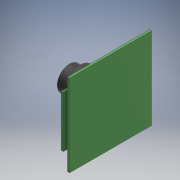
# Autodesk Inventor part: learnbotCamara
Saved by Autodesk Inventor 2017 (Build 210142000, 142)
## iProperties
Part Number: learnbotCamara
Material: Genérico
Document SubType Name: Modeling
Designer: rober
Density: 1 g/cm^3
Appearance: Valor por defecto
Author: rober
Autodesk Inventor part; units mm, degrees
ref_plane "YZ Plane" through (0, 0, 0) normal (1, 0, 0) x (0, 1, 0)
ref_plane "XZ Plane" through (0, 0, 0) normal (0, 1, 0) x (-1, 0, 0)
ref_plane "XY Plane" through (0, 0, 0) normal (0, 0, 1) x (1, 0, 0)
sketch "Boceto1" plane through (0, 0, 0) normal (0, 0, 1) x (1, 0, 0)
  line L0 (-1.6, 1.6) -> (-1.6, 1.2)
  line L1 (-1.1, 1.2) -> (-1.1, 2.8)
  line L2 (-1.1, 2.8) -> (-0.9, 2.8)
  line L3 (-0.9, 2.8) -> (-0.9, 1.2)
  line L4 (-0.2, 0.75) -> (-0.2, 3.25)
  line L5 (-0.9, 2.6) -> (-0.2, 2.6)
  line L6 (-0.2, 3.25) -> (0, 3.25)
  line L7 (0, 0) -> (0, 4)
  line L8 (-0.2, 0.75) -> (0, 0.75)
  line L9 (-1.1, 1) -> (-1.1, 1.2)
  line L10 (-0.9, 1.2) -> (-0.9, 1)
  line L11 (-1.1, 1) -> (-0.9, 1)
  line L12 (-1.6, 1.2) -> (-1.1, 1.2)
  line L13 (-0.9, 1.2) -> (-0.2, 1.2)
  line L14 (-1.1, 2.6) -> (-1.6, 2.6)
  line L15 (0.3, 0) -> (0.3, 4)
  line L16 (0, 0) -> (0.1, 0)
  line L17 (0.1, 0) -> (0.1, 4)
  line L18 (0.1, 4) -> (0, 4)
  line L19 (0.3, 0) -> (0.4, 0)
  line L20 (0.4, 0) -> (0.4, 4)
  line L21 (0.4, 4) -> (0.3, 4)
  line L22 (-1.6, 1.6) -> (-1.5, 1.6)
  line L23 (-1.5, 1.6) -> (-1.5, 2.2)
  line L24 (-1.5, 2.2) -> (-1.6, 2.2)
  line L25 (-1.6, 2.2) -> (-1.6, 2.6)
  constraints: 52 end point, 6 point on line
extrude "Extrusión1" add sketch "Boceto1" along normal blind 4 contours L7 L18 L17 L16 | L15 L21 L20 L19
sketch "Boceto2" plane through (0, 0, 0) normal (-1, 0, 0) x (0, 0, 1)
  line L0 (0, 4) -> (0, 0) projected
  line L1 (0, 0) -> (4, 0) projected
  line L2 (4, 4) -> (4, 0) projected
  line L3 (0, 4) -> (4, 4) projected
  line L4 (0, 4) -> (4, 4)
  line L5 (4, 0) -> (0, 0)
  line L6 (0, 0) -> (0, 4)
  circle A0 centre (2, 2) radius 0.8
  circle A1 centre (2, 2) radius 0.35
  circle A2 centre (2, 2) radius 0.6
  line L7 (1.4, 1.2) -> (1.4, 1.4708)
  line L8 (1.4, 2.5292) -> (1.4, 2.8)
  line L9 (2.6, 2.8) -> (2.6, 2.5292)
  line L10 (2.6, 1.4708) -> (2.6, 1.2)
  line L11 (2.4395, 1.2) -> (1.5605, 1.2)
  line L12 (1.4, 1.2) -> (1.9377, 0.7718)
  line L13 (2.0623, 0.7718) -> (2.6, 1.2)
  circle A3 centre (2, 3.15) radius 0.1
  circle A4 centre (2, 0.85) radius 0.1
  line L14 (1.5605, 1.2) -> (1.9218, 0.9123)
  line L15 (2.4395, 1.2) -> (2.0782, 0.9123)
  line L16 (2.4395, 2.8) -> (1.5605, 2.8)
  line L17 (1.5605, 2.8) -> (1.9218, 3.0877)
  line L18 (2.4395, 2.8) -> (2.0782, 3.0877)
  line L19 (1.4, 2.8) -> (1.9377, 3.2282)
  line L20 (2.0623, 3.2282) -> (2.6, 2.8)
  line L21 (0.75, 0) -> (0.75, 4)
  line L22 (0.75, 4) -> (3.25, 4)
  line L23 (3.25, 4) -> (3.25, 0)
  line L24 (4, 0) -> (4, 4)
  constraints: 42 end point, 12 point on circle, 5 centre point, 4 point on line
extrude "Extrusión2" cut sketch "Boceto2" against normal blind 0.2 contours L3 L21 L1 L0 | L3 L2 L1 L23
sketch "Boceto3" plane through (0, 0, 0.75) normal (-1, 0, 0) x (0, 0, 1)
  line L0 (-0.75, 4) -> (3.25, 4)
  line L1 (3.25, 0) -> (-0.75, 0)
  line L2 (-0.75, 0) -> (-0.75, 4)
  circle A0 centre (1.25, 2) radius 0.8
  circle A1 centre (1.25, 2) radius 0.35
  circle A2 centre (1.25, 2) radius 0.6
  line L3 (0.65, 1.2) -> (0.65, 1.4708)
  line L4 (0.65, 2.5292) -> (0.65, 2.8)
  line L5 (1.85, 2.8) -> (1.85, 2.5292)
  line L6 (1.85, 1.4708) -> (1.85, 1.2)
  line L7 (1.6895, 1.2) -> (0.8105, 1.2)
  line L8 (0.65, 1.2) -> (1.1877, 0.7718)
  line L9 (1.3123, 0.7718) -> (1.85, 1.2)
  circle A3 centre (1.25, 3.15) radius 0.1
  circle A4 centre (1.25, 0.85) radius 0.1
  line L10 (0.8105, 1.2) -> (1.1718, 0.9123)
  line L11 (1.6895, 1.2) -> (1.3282, 0.9123)
  line L12 (1.6895, 2.8) -> (0.8105, 2.8)
  line L13 (0.8105, 2.8) -> (1.1718, 3.0877)
  line L14 (1.6895, 2.8) -> (1.3282, 3.0877)
  line L15 (0.65, 2.8) -> (1.1877, 3.2282)
  line L16 (1.3123, 3.2282) -> (1.85, 2.8)
  line L17 (0, 0) -> (0, 4)
  line L18 (0, 4) -> (2.5, 4)
  line L19 (2.5, 4) -> (2.5, 0)
  line L20 (3.25, 0) -> (3.25, 4)
  line L21 (0, 4) -> (0, 0) projected
  line L22 (0, 0) -> (2.5, 0) projected
  line L23 (2.5, 0) -> (2.5, 4) projected
  line L24 (0, 4) -> (2.5, 4) projected
  constraints: 42 end point, 12 point on circle, 5 centre point, 4 point on line
extrude "Extrusión3" add sketch "Boceto3" along normal blind 0.2 contours A0 | A0 L12 L14 A3 L16 L5 | L6 L9 A4 L11 L7 A0 | A0 L4 L15 A3 L13 L12 | L7 L10 A4 L8 L3 A0 | A3 | A4 | A1 | A2
sketch "Boceto4" plane through (-0.2, 0, 0.75) normal (-1, 0, 0) x (0, 0, 1)
  line L0 (-0.75, 4) -> (3.25, 4)
  line L1 (3.25, 0) -> (-0.75, 0)
  line L2 (-0.75, 0) -> (-0.75, 4)
  circle A0 centre (1.25, 2) radius 0.8
  circle A1 centre (1.25, 2) radius 0.35
  circle A2 centre (1.25, 2) radius 0.6
  line L3 (0.65, 1.2) -> (0.65, 1.4708)
  line L4 (0.65, 2.5292) -> (0.65, 2.8)
  line L5 (1.85, 2.8) -> (1.85, 2.5292)
  line L6 (1.85, 1.4708) -> (1.85, 1.2)
  line L7 (1.6895, 1.2) -> (0.8105, 1.2)
  line L8 (0.65, 1.2) -> (1.1877, 0.7718)
  line L9 (1.3123, 0.7718) -> (1.85, 1.2)
  circle A3 centre (1.25, 3.15) radius 0.1
  circle A4 centre (1.25, 0.85) radius 0.1
  line L10 (0.8105, 1.2) -> (1.1718, 0.9123)
  line L11 (1.6895, 1.2) -> (1.3282, 0.9123)
  line L12 (1.6895, 2.8) -> (0.8105, 2.8)
  line L13 (0.8105, 2.8) -> (1.1718, 3.0877)
  line L14 (1.6895, 2.8) -> (1.3282, 3.0877)
  line L15 (0.65, 2.8) -> (1.1877, 3.2282)
  line L16 (1.3123, 3.2282) -> (1.85, 2.8)
  line L17 (0, 0) -> (0, 4)
  line L18 (0, 4) -> (2.5, 4)
  line L19 (2.5, 4) -> (2.5, 0)
  line L20 (3.25, 0) -> (3.25, 4)
  line L21 (1.6895, 2.8) -> (0.8105, 2.8) projected
  line L22 (0.8105, 2.8) -> (1.1718, 3.0877) projected
  arc A5 (1.1718, 3.0877) -> (1.3282, 3.0877) centre (1.25, 3.15) ccw projected
  line L23 (1.3282, 3.0877) -> (1.6895, 2.8) projected
  line L24 (1.6895, 1.2) -> (1.3282, 0.9123) projected
  arc A6 (1.3282, 0.9123) -> (1.1718, 0.9123) centre (1.25, 0.85) ccw projected
  line L25 (1.1718, 0.9123) -> (0.8105, 1.2) projected
  line L26 (0.8105, 1.2) -> (1.6895, 1.2) projected
  line L27 (0.65, 1.2) -> (1.1877, 0.7718) projected
  arc A7 (1.1877, 0.7718) -> (1.3123, 0.7718) centre (1.25, 0.85) ccw projected
  line L28 (1.3123, 0.7718) -> (1.85, 1.2) projected
  line L29 (1.85, 1.2) -> (1.85, 1.4708) projected
  arc A8 (1.85, 1.4708) -> (1.85, 2.5292) centre (1.25, 2) ccw projected
  line L30 (1.85, 2.5292) -> (1.85, 2.8) projected
  line L31 (1.85, 2.8) -> (1.3123, 3.2282) projected
  arc A9 (1.3123, 3.2282) -> (1.1877, 3.2282) centre (1.25, 3.15) ccw projected
  line L32 (1.1877, 3.2282) -> (0.65, 2.8) projected
  line L33 (0.65, 2.8) -> (0.65, 2.5292) projected
  arc A10 (0.65, 2.5292) -> (0.65, 1.4708) centre (1.25, 2) ccw projected
  line L34 (0.65, 1.4708) -> (0.65, 1.2) projected
  point P0 (-0.75, 0)
  constraints: 42 end point, 12 point on circle, 5 centre point, 4 point on line
extrude "Extrusión4" add sketch "Boceto4" along normal blind 0.7 contours A1 | A2
sketch "Boceto5" plane through (-0.9, 2, 2) normal (-1, 0, 0) x (0, 0, 1)
  line L0 (-2, 2) -> (2, 2)
  line L1 (2, -2) -> (-2, -2)
  line L2 (-2, -2) -> (-2, 2)
  circle A0 centre (0, 0) radius 0.8
  circle A1 centre (0, 0) radius 0.35
  circle A2 centre (0, 0) radius 0.6
  line L3 (-0.6, -0.8) -> (-0.6, -0.5292)
  line L4 (-0.6, 0.5292) -> (-0.6, 0.8)
  line L5 (0.6, 0.8) -> (0.6, 0.5292)
  line L6 (0.6, -0.5292) -> (0.6, -0.8)
  line L7 (0.4395, -0.8) -> (-0.4395, -0.8)
  line L8 (-0.6, -0.8) -> (-0.0623, -1.2282)
  line L9 (0.0623, -1.2282) -> (0.6, -0.8)
  circle A3 centre (0, 1.15) radius 0.1
  circle A4 centre (0, -1.15) radius 0.1
  line L10 (-0.4395, -0.8) -> (-0.0782, -1.0877)
  line L11 (0.4395, -0.8) -> (0.0782, -1.0877)
  line L12 (0.4395, 0.8) -> (-0.4395, 0.8)
  line L13 (-0.4395, 0.8) -> (-0.0782, 1.0877)
  line L14 (0.4395, 0.8) -> (0.0782, 1.0877)
  line L15 (-0.6, 0.8) -> (-0.0623, 1.2282)
  line L16 (0.0623, 1.2282) -> (0.6, 0.8)
  line L17 (-1.25, -2) -> (-1.25, 2)
  line L18 (-1.25, 2) -> (1.25, 2)
  line L19 (1.25, 2) -> (1.25, -2)
  line L20 (2, -2) -> (2, 2)
  circle A5 centre (0, 0) radius 0.6 projected
  point P0 (-2, -2)
  constraints: 42 end point, 12 point on circle, 5 centre point, 4 point on line
extrude "Extrusión5" add sketch "Boceto5" along normal blind 0.2 contours A0 | A1 | A2
sketch "Boceto6" plane through (-1.1, 2, 2) normal (-1, 0, 0) x (0, 0, 1)
  line L0 (-2, 2) -> (2, 2)
  line L1 (2, -2) -> (-2, -2)
  line L2 (-2, -2) -> (-2, 2)
  circle A0 centre (0, 0) radius 0.8
  circle A1 centre (0, 0) radius 0.35
  circle A2 centre (0, 0) radius 0.6
  line L3 (-0.6, -0.8) -> (-0.6, -0.5292)
  line L4 (-0.6, 0.5292) -> (-0.6, 0.8)
  line L5 (0.6, 0.8) -> (0.6, 0.5292)
  line L6 (0.6, -0.5292) -> (0.6, -0.8)
  line L7 (0.4395, -0.8) -> (-0.4395, -0.8)
  line L8 (-0.6, -0.8) -> (-0.0623, -1.2282)
  line L9 (0.0623, -1.2282) -> (0.6, -0.8)
  circle A3 centre (0, 1.15) radius 0.1
  circle A4 centre (0, -1.15) radius 0.1
  line L10 (-0.4395, -0.8) -> (-0.0782, -1.0877)
  line L11 (0.4395, -0.8) -> (0.0782, -1.0877)
  line L12 (0.4395, 0.8) -> (-0.4395, 0.8)
  line L13 (-0.4395, 0.8) -> (-0.0782, 1.0877)
  line L14 (0.4395, 0.8) -> (0.0782, 1.0877)
  line L15 (-0.6, 0.8) -> (-0.0623, 1.2282)
  line L16 (0.0623, 1.2282) -> (0.6, 0.8)
  line L17 (-1.25, -2) -> (-1.25, 2)
  line L18 (-1.25, 2) -> (1.25, 2)
  line L19 (1.25, 2) -> (1.25, -2)
  line L20 (2, -2) -> (2, 2)
  circle A5 centre (0, 0) radius 0.8 projected
  point P0 (-2, -2)
  constraints: 42 end point, 12 point on circle, 5 centre point, 4 point on line
extrude "Extrusión6" add sketch "Boceto6" along normal blind 0.5 contours A1 | A2
sketch "Boceto7" plane through (-1.6, 2, 2) normal (-1, 0, 0) x (0, 0, 1)
  circle A0 centre (0, 0) radius 0.6 projected
  circle A1 centre (0, 0) radius 0.3
  point P0 (-2, -2)
  dimension "d12" = 0.6
  constraints: 1 centre point, 1 coincident
  measures "d12" diameter of A1
extrude "Extrusión7" cut sketch "Boceto7" against normal blind 0.1 contours A1
